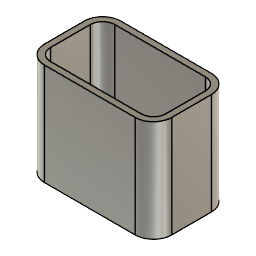
▢-125×75×6.0 (Autodesk Fusion 360 design; units mm, degrees)
Autodesk Fusion 360 part; units mm, degrees
sketch "スケッチ1" plane through (0, 0, 0) normal (0, 0, 1) x (1, 0, 0)
  arc A0 (448.7951, 143.9553) -> (466.7951, 161.9553) centre (448.7951, 161.9553) ccw
  arc A1 (448.7951, 149.9553) -> (460.7951, 161.9553) centre (448.7951, 161.9553) ccw
  arc A2 (341.7951, 161.9553) -> (359.7951, 143.9553) centre (359.7951, 161.9553) ccw
  arc A3 (347.7951, 161.9553) -> (359.7951, 149.9553) centre (359.7951, 161.9553) ccw
  line L0 (359.7951, 143.9553) -> (448.7951, 143.9553)
  line L1 (359.7951, 149.9553) -> (448.7951, 149.9553)
  line L2 (448.7951, 218.9553) -> (359.7951, 218.9553)
  line L3 (448.7951, 212.9553) -> (359.7951, 212.9553)
  line L4 (341.7951, 200.9553) -> (341.7951, 161.9553)
  line L5 (347.7951, 200.9553) -> (347.7951, 161.9553)
  arc A4 (359.7951, 218.9553) -> (341.7951, 200.9553) centre (359.7951, 200.9553) ccw
  arc A5 (359.7951, 212.9553) -> (347.7951, 200.9553) centre (359.7951, 200.9553) ccw
  line L6 (466.7951, 161.9553) -> (466.7951, 200.9553)
  line L7 (460.7951, 161.9553) -> (460.7951, 200.9553)
  arc A6 (466.7951, 200.9553) -> (448.7951, 218.9553) centre (448.7951, 200.9553) ccw
  arc A7 (460.7951, 200.9553) -> (448.7951, 212.9553) centre (448.7951, 200.9553) ccw
  point P0 (404.2951, 181.4553)
extrude "押し出し1" add sketch "スケッチ1" along normal blind 100
